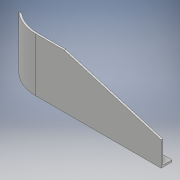
# Autodesk Inventor part: endplate_ver2
Saved by Autodesk Inventor 2018 (Build 220112000, 112)
## iProperties
Created: 2018-05-11
Part Number: endplate_ver2
Material: 一般
Document SubType Name: Modeling
Designer: ku_sk
Density: 1 g/cm^3
Appearance: 既定
Author: ku_sk
Autodesk Inventor part; units mm, degrees
ref_plane "YZ Plane" through (0, 0, 0) normal (1, 0, 0) x (0, 1, 0)
ref_plane "XZ Plane" through (0, 0, 0) normal (0, 1, 0) x (-1, 0, 0)
ref_plane "XY Plane" through (0, 0, 0) normal (0, 0, 1) x (1, 0, 0)
sketch "スケッチ1" plane through (0, 0, 0) normal (0, 1, 0) x (-1, 0, 0)
  line L0 (250, 100) -> (-250, 100)
  line L1 (-250, 100) -> (-250, -100)
  line L2 (-250, -100) -> (250, -100)
  line L3 (250, -100) -> (250, 100)
  point P0 (0, 0)
  dimension "d2" = 250
  dimension "d3" = 500
  dimension "d4" = 100
  dimension "d5" = 200
  constraints: 8 end point, 2 parallel, 1 horizontal, 1 perpendicular
  measures "d2" distance from line of point (0, 0) L3
  measures "d3" distance of L0.start L0.end
  measures "d4" distance from line of point (0, 0) L0
  measures "d5" distance of L2.end L0.start
extrude "押し出し1" add sketch "スケッチ1" along normal blind 35
sketch "スケッチ2" plane through (-250, 0, 100) normal (0, 0, 1) x (1, 0, 0)
  line L0 (0, 35) -> (500, 35) projected
  line L1 (0, 0) -> (500, 0) projected
  arc A0 (0, 35) -> (90, 0) centre (90, 133.2143) ccw
  line L2 (0, 0) -> (0, 35) projected
  point P0 (250, 0)
  dimension "d8" = 90
  constraints: 2 point on circle, 1 centre point, 1 point on line, 1 tangent
  measures "d8" distance from line of L2 A0.end
extrude "押し出し2" cut sketch "スケッチ2" against normal through all
sketch "スケッチ5" plane through (-160, 0, 100) normal (0, 0, 1) x (1, 0, 0)
  arc A0 (-90, 35) -> (0, 0) centre (0, 133.2143) ccw projected
  line L0 (0, 0) -> (410, 0) projected
  arc A1 (-80.8544, 35) -> (0, 6) centre (0, 133.2143) ccw
  line L1 (0, 6) -> (54.4195, 6)
  line L2 (54.4195, 6) -> (410, 6)
  line L3 (-90, 35) -> (410, 35) projected
  line L4 (410, 0) -> (410, 35) projected
  point P0 (160, 0)
  point P1 (40, 35)
  dimension "d20" = 6
  constraints: 4 end point, 2 point on circle, 1 centre point, 1 collinear, 1 point on line, 1 other
  measures "d20" radial gap between concentric circles of A0 A1
extrude "押し出し5" cut sketch "スケッチ5" against normal through all contours L3 L4 L2 L1 A1
sketch "スケッチ8" plane through (-160, 6, 100) normal (0, 1, 0) x (1, 0, 0)
  line L0 (210, 150) -> (160, 150)
  line L1 (410, 200) -> (410, 0) projected
  line L2 (0, 200) -> (410, 200) projected
  arc A0 (160, 150) -> (-90, 80) centre (160, -331.4286) ccw
  line L3 (-90, 200) -> (-90, 0) projected
  line L4 (-80.8544, 200) -> (0, 200) projected
  line L5 (-80.8544, 200) -> (-90, 200) projected
  line L6 (210, 156) -> (160, 156)
  arc A1 (160, 156) -> (-90, 87.005) centre (160, -331.4286) ccw
  line L7 (210, 150) -> (210, 156)
  line L8 (410, 0) -> (410, 200) projected
  line L9 (-90, 87.005) -> (-90, 80)
  point P0 (160, 100)
  dimension "d35" = 50
  dimension "d36" = 120
  dimension "d38" = 6
  dimension "d47" = 250
  dimension "d48" = 50
  constraints: 8 end point, 4 point on circle, 2 centre point, 2 point on line, 1 horizontal, 1 parallel, 1 tangent, 1 vertical, 2 other
  measures "d35" distance between parallel lines of L2 L0
  measures "d36" distance from line of L9.end L2
  measures "d38" distance between parallel lines of L0 L6
  measures "d47" distance from line of L3 L6.end
  measures "d48" distance of L6.start L6.end
extrude "押し出し7" add sketch "スケッチ8" along normal up to surface (29 mm away)
delete faces "面を削除1" heal yes whole lump no faces at (-246.2129, 22.2141, 17.7225) (-250, 25.3333, 15.33) (-244.511, 6, 14.4766) (-246.2115, 22.2135, 10.7547)
sketch "スケッチ10" plane through (-160, 6, 100) normal (0, 1, 0) x (1, 0, 0)
  line L0 (410, 150) -> (410, 0) projected
  line L1 (410, 0) -> (0, 0) projected
  line L2 (410, 0) -> (410, 200) projected
  line L3 (410, 120) -> (10, 0)
  line L4 (0, 0) -> (410, 0) projected
  point P0 (160, 100)
  point P1 (210, 150)
  dimension "d43" = 400
  dimension "d44" = 120
  constraints: 2 end point, 2 point on line, 4 other
  measures "d44" distance from line of L3.start L1
extrude "押し出し9" cut sketch "スケッチ10" against normal through all
sketch "スケッチ11" plane through (250, 6, -100) normal (0, 0, -1) x (-1, 0, 0)
  line L0 (0, -6) -> (410, -6) projected
  arc A0 (410, -6) -> (500, 29) centre (410, 127.2143) ccw projected
  line L1 (0, -6) -> (0, 29)
  line L2 (0, 29) -> (500, 29)
  point P0 (250, -6)
  constraints: 4 end point, 1 perpendicular, 1 vertical
extrude "押し出し10" add sketch "スケッチ11" against normal blind 6
sketch "スケッチ12" plane through (0, 0, 0) normal (0, 1, 0) x (-1, 0, 0)
  line L0 (250, -100) -> (250, 100) projected
  line L1 (250, 100) -> (0, 100)
  line L2 (0, 100) -> (0, 75)
  line L3 (0, 75) -> (250, 75)
  line L4 (250, 75) -> (250, 100)
  point P0 (0, 0)
  dimension "d51" = 25
  constraints: 8 end point, 2 parallel, 1 horizontal, 1 perpendicular
  measures "d51" distance of L1.end L2.end
extrude "押し出し11" cut sketch "スケッチ12" along normal through all
